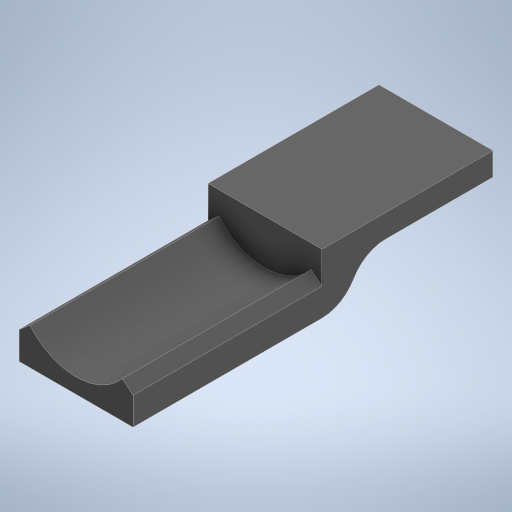
# Autodesk Inventor part: arm_1_remake
Saved by Autodesk Inventor 2024.1 (Build 281209000, 209)
## iProperties
Created: 2025-01-27
Part Number: arm_1_remake
Material: 一般
Document SubType Name: Modeling
Designer: hibik
Density: 1 g/cm^3
Appearance: 既定
Author: hibik
Autodesk Inventor part; units mm, degrees
ref_plane "YZ Plane" through (0, 0, 0) normal (1, 0, 0) x (0, 1, 0)
ref_plane "XZ Plane" through (0, 0, 0) normal (0, 1, 0) x (-1, 0, 0)
ref_plane "XY Plane" through (0, 0, 0) normal (0, 0, 1) x (1, 0, 0)
sketch "スケッチ1" plane through (0, 0, 0) normal (0, 1, 0) x (-1, 0, 0)
  line L0 (11.25, 0) -> (-11.25, 0)
  line L1 (-11.25, 0) -> (-11.25, -120)
  line L2 (-11.25, -120) -> (11.25, -120)
  line L3 (11.25, -120) -> (11.25, 0)
  point P0 (0, 0)
  point P1 (0, 0)
  dimension "d0" = 22.5
  dimension "d3" = 120
  constraints: 8 end point, 2 parallel, 1 coincident, 1 horizontal, 1 midpoint, 1 perpendicular
  measures "d0" distance of L0.start L0.end
  measures "d3" distance of L2.end L0.start
extrude "押し出し1" add sketch "スケッチ1" along normal blind 2
sketch "スケッチ2" plane through (0, 0, 0) normal (0, -1, 0) x (1, 0, 0)
  line L0 (19, -120) -> (-19, -120)
  line L1 (-19, -120) -> (-19, -103.05)
  line L2 (-19, -103.05) -> (19, -103.05)
  line L3 (19, -103.05) -> (19, -120)
  line L4 (11.25, -120) -> (-11.25, -120) projected
  point P0 (0, 0)
  point P1 (0, -120)
  dimension "d6" = 38
  dimension "d11" = 16.95
  constraints: 8 end point, 2 midpoint, 2 parallel, 1 collinear, 1 horizontal, 1 perpendicular
  measures "d6" distance of L0.start L0.end
  measures "d11" distance of L0.end L1.end
extrude "押し出し2" add sketch "スケッチ2" against normal blind 13.44
sketch "スケッチ4" plane through (11.25, 0, -103.05) normal (0, 0, 1) x (1, 0, 0)
  circle A0 centre (-11.25, 20) radius 20
  line L0 (7.75, 0) -> (0, 0) projected
  line L1 (-22.5, 0) -> (0, 0) projected
  point P0 (-11.25, 0)
  point P1 (-11.25, 0)
  dimension "d12" = 40
  constraints: 1 centre point, 1 midpoint, 1 tangent, 1 vertical alignment
  measures "d12" diameter of A0
extrude "押し出し4" cut sketch "スケッチ4" along normal through all
sketch "スケッチ5" plane through (11.25, 0, -103.05) normal (0, 0, 1) x (1, 0, 0)
  circle A0 centre (-11.25, 20) radius 20
  arc A1 (-11.25, 0) -> (-2.5322, 2) centre (-11.25, 20) ccw projected
  line L0 (-30.25, 13.44) -> (7.75, 13.44)
  line L1 (7.75, 13.44) -> (7.75, -5)
  line L2 (7.75, -5) -> (-30.25, -5)
  line L3 (-30.25, -5) -> (-30.25, 13.44)
  line L4 (7.75, 0) -> (7.75, 13.44) projected
  line L5 (7.75, 0) -> (0, 0) projected
  line L6 (-30.25, 4.22) -> (-11.25, 20)
  line L7 (-11.25, 20) -> (7.75, 4.22)
  point P0 (3.875, 0)
  point P1 (7.6436, 13.44)
  point P2 (-30.1436, 13.44)
  point P3 (7.75, 4.22)
  point P4 (4.1356, 7.2218)
  point P5 (-26.6356, 7.2218)
  point P6 (-3.3514, 13.44)
  point P7 (-19.1486, 13.44)
  dimension "d15" = 5
  constraints: 12 end point, 3 midpoint, 2 concentric, 2 parallel, 1 centre point, 1 collinear, 1 horizontal, 1 horizontal alignment, 1 perpendicular, 1 point on line
  measures "d15" distance from line of L2 point (3.875, 0)
extrude "押し出し5" add sketch "スケッチ5" along normal up to surface (103.05 mm away) contours A0 L7 L1 L2 L3 L6
sketch "スケッチ24" plane through (11.25, 0, -103.05) normal (0, 0, -1) x (-1, 0, 0)
  line L0 (-7.75, 0) -> (11.25, 0) projected
  line L1 (-7.75, -5) -> (-7.75, 0) projected
  line L2 (30.25, -5) -> (-7.75, -5) projected
  line L3 (30.25, 0) -> (30.25, -5) projected
  line L4 (11.25, 0) -> (30.25, 0) projected
  point P0 (11.25, 0)
extrude "押し出し22" add sketch "スケッチ24" along normal up to surface (16.95 mm away)
sketch "スケッチ25" plane through (19, 13.44, -103.05) normal (1, 0, 0) x (0, 0, -1)
  line L0 (-103.05, -13.44) -> (-103.05, -6.2182) projected
  line L1 (16.95, -18.44) -> (16.95, 0) projected
  line L2 (16.95, -13.44) -> (-40.05, -13.44)
  line L3 (-40.05, -13.44) -> (-40.05, 1.46)
  line L4 (-40.05, 1.46) -> (16.95, 1.46)
  line L5 (16.95, 1.46) -> (16.95, -13.44)
  dimension "d77" = 14.9
  dimension "d78" = 57
  constraints: 8 end point, 2 parallel, 2 point on line, 1 horizontal, 1 perpendicular
  measures "d77" distance of L4.end L2.start
  measures "d78" distance of L3.end L4.end
extrude "押し出し23" add sketch "スケッチ25" against normal up to surface (38 mm away)
sketch "スケッチ26" plane through (19, -5, 0) normal (1, 0, 0) x (0, 0, -1)
  line L0 (63, 12.2218) -> (0, 12.2218) projected
  circle A0 centre (63, 12.2218) radius 12.2218
  line L1 (0, 0) -> (120, 0) projected
  circle A1 centre (84.1688, 0) radius 12.2218
  line L2 (84.1688, 12.2218) -> (120, 12.2218)
  line L3 (120, 0) -> (120, 19.9) projected
  point P0 (0, 5)
  point P1 (73.5844, 6.1109)
  point P2 (63, 0)
  constraints: 2 end point, 2 horizontal, 2 point on line, 1 centre point, 1 coincident, 1 tangent, 5 other
extrude "押し出し24" cut sketch "スケッチ26" against normal through all contours A1 L1 A0 | A1 L1 | L2 L3 L1 A1 picked at (80.2991, 4.512)
